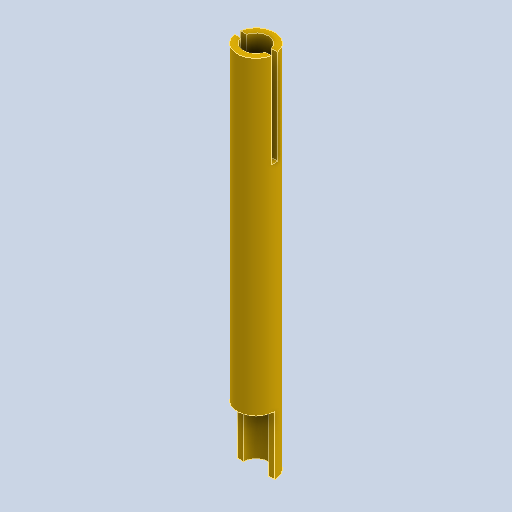
# Autodesk Inventor part: SMA-PanelMount-Ni-AuPlated-Pin
Saved by Autodesk Inventor 2026 (Build 300175050, 175E)
## iProperties
Created: 2026-02-17
Part Number: SMA-PanelMount-Ni-AuPlated-Pin
Material: Brass
Document SubType Name: Modeling
Designer: schanen
Density: 8.49 g/cm^3
Appearance: Gold
Author: schanen
Autodesk Inventor part; units mm, degrees
ref_plane "YZ Plane" through (0, 0, 0) normal (1, 0, 0) x (0, 1, 0)
ref_plane "XZ Plane" through (0, 0, 0) normal (0, 1, 0) x (-1, 0, 0)
ref_plane "XY Plane" through (0, 0, 0) normal (0, 0, 1) x (1, 0, 0)
sketch "Sketch1" plane through (0, 0, 0) normal (0, 0, 1) x (1, 0, 0)
  line L0 (0, 9.3) -> (-0.425, 9.3)
  line L1 (-0.425, 9.3) -> (-0.425, 12.5)
  line L2 (-0.425, 12.5) -> (-0.635, 12.5)
  line L3 (-0.635, 12.5) -> (-0.635, 0)
  line L4 (-0.635, 0) -> (-0.425, 0)
  line L5 (-0.425, 0) -> (-0.425, 4)
  line L6 (-0.425, 4) -> (0, 4)
  line L7 (0, 4) -> (0, 9.3)
  point P0 (0, 0)
  dimension "d0" = 0.635
  dimension "d1" = 12.5
  dimension "d2" = 4
  dimension "d3" = 3.2
  dimension "d4" = 0.425
  constraints: 16 end point, 7 perpendicular, 2 vertical alignment, 1 horizontal, 1 horizontal alignment
  measures "d0" distance from line of point (0, 0) L3
  measures "d1" distance of L2.end L3.end
  measures "d2" distance of L4.end L5.end
  measures "d3" distance of L0.end L1.end
  measures "d4" distance between parallel lines of L7 L1
revolve "Revolution1" add sketch "Sketch1" angle 360 about axis through (0, 4, 0) along (0, 1, 0)
sketch "Sketch2" plane through (0, 0, 0) normal (1, 0, 0) x (0, 1, 0)
  line L0 (9.3, -0.425) -> (9.3, 0.425) projected
  line L1 (9.3, -0.1) -> (12.5, -0.1)
  line L2 (12.5, -0.425) -> (12.5, 0.425) projected
  line L3 (9.3, 0.1) -> (12.5, 0.1)
  line L4 (9.3, -0.1) -> (9.3, 0.1)
  line L5 (12.5, -0.1) -> (12.5, 0.1)
  point P0 (0, 0)
  dimension "d6" = 0.2
  dimension "d7" = 0.1
  constraints: 8 end point, 4 point on line, 2 perpendicular, 1 collinear, 1 horizontal
  measures "d6" distance between parallel lines of L3 L1
  measures "d7" distance from line of point (0, 0) L1
extrude "Extrusion1" cut sketch "Sketch2" along normal through all both and the other way through all
sketch "Sketch3" plane through (0, 0, 0) normal (1, 0, 0) x (0, 1, 0)
  line L0 (0, 0) -> (2, 0)
  line L1 (0, 0.635) -> (12.5, 0.635) projected
  line L2 (2, 0) -> (2, 0.635)
  line L3 (0, -0.635) -> (0, 0.635) projected
  line L4 (0, 0) -> (0, 0.635)
  line L5 (2, 0.635) -> (0, 0.635)
  dimension "d10" = 2
  constraints: 8 end point, 1 collinear, 1 horizontal, 1 perpendicular, 1 point on line, 1 vertical
  measures "d10" distance of L0.start L0.end
extrude "Extrusion2" cut sketch "Sketch3" along normal through all both and the other way through all
body "Solid1"
